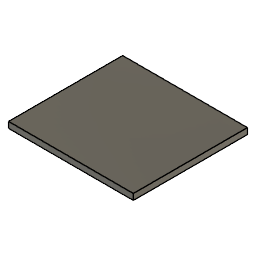
ultra schuin (Autodesk Fusion 360 design; units mm, degrees)
part number: 2026-03-26-09-14-51-518
Autodesk Fusion 360 part; units mm, degrees
sketch "Sketch1" plane through (0, 0, 0) normal (0, 0, 1) x (1, 0, 0)
  line L0 (-7.9973, 42.0732) -> (74.0027, 42.0732)
  line L1 (74.0027, 42.0732) -> (74.0027, -12.9268)
  line L2 (74.0027, -12.9268) -> (-7.9973, -12.9268)
  line L3 (-7.9973, -12.9268) -> (-7.9973, 42.0732)
  constraint horizontal L0
  constraint vertical L1
  constraint horizontal L2
  constraint vertical L3
extrude "Extrude1" add sketch "Sketch1" along normal blind 4
extrude "Extrude2" add 1 faces at (46.6694, -12.9268, 1.3333) along direction (0, -1, 0) blind 15
extrude "Extrude3" add 1 faces at (46.6694, -27.9268, 1.3333) along direction (0, -1, 0) blind 5
